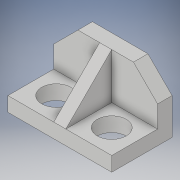
# Autodesk Inventor part: 410571040-T2
Saved by Autodesk Inventor 2017 (Build 210142000, 142)
## iProperties
Part Number: 410571040-T2
Material: 一般
Document SubType Name: Modeling
Designer: user
Density: 1 g/cm^3
Appearance: 預設
Author: user
Autodesk Inventor part; units mm, degrees
ref_plane "YZ Plane" through (0, 0, 0) normal (1, 0, 0) x (0, 1, 0)
ref_plane "XZ Plane" through (0, 0, 0) normal (0, 1, 0) x (-1, 0, 0)
ref_plane "XY Plane" through (0, 0, 0) normal (0, 0, 1) x (1, 0, 0)
sketch "草圖1" plane through (0, 0, 0) normal (0, 0, 1) x (1, 0, 0)
  line L0 (0, 0) -> (0, 15)
  line L1 (0, 15) -> (-10, 25)
  line L2 (-10, 25) -> (-33, 25)
  line L3 (-33, 25) -> (-43, 15)
  line L4 (-43, 15) -> (-43, 0)
  line L5 (-43, 0) -> (0, 0)
  dimension "d0" = 10
  dimension "d1" = 10
  dimension "d2" = 43
  dimension "d3" = 25
  dimension "d4" = 10
  constraints: 12 end point, 3 perpendicular, 1 parallel, 1 vertical
  measures "d0" horizontal distance of L0.end L1.end
  measures "d1" horizontal distance of L0.end L1.end
  measures "d2" distance of L4.end L0.start
  measures "d3" distance between parallel lines of L2 L5
  measures "d4" horizontal distance of L3.end L2.end
extrude "擠出1" add sketch "草圖1" against normal blind 6
sketch "草圖2" plane through (0, 0, 0) normal (1, 0, 0) x (0, 0, -1)
  line L0 (0, 0) -> (0, 15) projected
  line L1 (0, 6) -> (-19, 6)
  line L2 (-19, 6) -> (-19, 0)
  line L3 (0, 0) -> (6, 0) projected
  line L4 (-19, 0) -> (0, 0)
  line L5 (0, 0) -> (0, 6)
  dimension "d7" = 6
  dimension "d8" = 19
  constraints: 8 end point, 4 perpendicular, 1 point on line
  measures "d7" distance of L1.end L2.end
  measures "d8" distance between parallel lines of L2 L0
extrude "擠出2" add sketch "草圖2" against normal blind 43
ref_plane "工作平面1" through (-21.5, 0, -6) normal (1, 0, 0) x (0, 0, -1)
sketch "草圖3" plane through (-21.5, 0, -6) normal (1, 0, 0) x (0, 0, -1)
  line L0 (-25, 6) -> (-25, 0) projected
  line L1 (-25, 6) -> (-6, 25)
  line L2 (-6, 15) -> (-6, 6) projected
  line L3 (-6, 6) -> (-25, 6) projected
  point P0 (-6, 0)
  dimension "d12" = 19
  constraints: 2 end point, 1 point on line
  measures "d12" distance from line of L3 L1.end
extrude "肋1" add sketch "草圖3" along normal mid plane 5 rib yes fills toward (-15.4646, 15.4646) open curves L1
sketch "草圖4" plane through (-43, 6, 19) normal (0, 1, 0) x (1, 0, 0)
  circle A0 centre (10, 10) radius 6
  circle A1 centre (33, 10) radius 6
  line L0 (0, 0) -> (0, 19) projected
  line L1 (19, 0) -> (0, 0) projected
  line L2 (43, 0) -> (24, 0) projected
  line L3 (43, 19) -> (43, 0) projected
  dimension "d19" = 12
  dimension "d20" = 10
  dimension "d21" = 10
  dimension "d22" = 10
  dimension "d23" = 10
  dimension "d24" = 12
  constraints: 2 centre point
  measures "d19" diameter of A1
  measures "d20" distance from line of A0.centre L0
  measures "d21" distance from line of A0.centre L1
  measures "d22" distance from line of A1.centre L2
  measures "d23" distance from line of A1.centre L3
  measures "d24" diameter of A0
extrude "擠出3" cut sketch "草圖4" against normal blind 43
